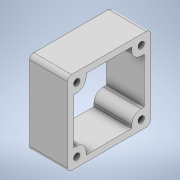
# Autodesk Inventor part: encoder_cover
Saved by Autodesk Inventor 2021 (Build 250183000, 183)
## iProperties
Created: 2021-01-13
Part Number: encoder_cover
Material: Generic
Document SubType Name: Modeling
Designer: Mateusz
Density: 1 g/cm^3
Appearance: Default
Author: Mateusz
Autodesk Inventor part; units mm, degrees
ref_plane "YZ Plane" through (0, 0, 0) normal (1, 0, 0) x (0, 1, 0)
ref_plane "XZ Plane" through (0, 0, 0) normal (0, 1, 0) x (-1, 0, 0)
ref_plane "XY Plane" through (0, 0, 0) normal (0, 0, 1) x (1, 0, 0)
sketch "Sketch1" plane through (0, 0, 0) normal (1, 0, 0) x (0, 1, 0)
  circle A0 centre (0, 0) radius 1.45
  circle A1 centre (0, -31) radius 1.45
  circle A2 centre (-31, -31) radius 1.45
  circle A3 centre (-31, 0) radius 1.45
  line L0 (0, 4.5) -> (-31, 4.5)
  line L1 (-31, 4.5) -> (-35.5, 4.5)
  line L2 (-35.5, 4.5) -> (-35.5, -35.5)
  line L3 (-35.5, -35.5) -> (4.5, -35.5)
  line L4 (4.5, -35.5) -> (4.5, 4.5)
  line L5 (4.5, 4.5) -> (0, 4.5)
  arc A4 (-4.5, 0) -> (0, -4.5) centre (0, 0) ccw
  arc A5 (-26.5, -31) -> (-31, -26.5) centre (-31, -31) ccw
  line L6 (-26.5, 0) -> (-26.5, 1.5)
  line L7 (-31, -4.5) -> (-32.5, -4.5)
  line L8 (-31, -26.5) -> (-32.5, -26.5)
  line L9 (-26.5, -31) -> (-26.5, -32.5)
  line L10 (-4.5, -31) -> (-4.5, -32.5)
  line L11 (0, -26.5) -> (1.5, -26.5)
  line L12 (0, -4.5) -> (1.5, -4.5)
  line L13 (-4.5, 0) -> (-4.5, 1.5)
  arc A6 (0, -26.5) -> (-4.5, -31) centre (0, -31) ccw
  arc A7 (-31, -4.5) -> (-26.5, 0) centre (-31, 0) ccw
  line L14 (-26.5, 1.5) -> (-4.5, 1.5)
  line L15 (1.5, -4.5) -> (1.5, -26.5)
  line L16 (-4.5, -32.5) -> (-26.5, -32.5)
  line L17 (-32.5, -26.5) -> (-32.5, -4.5)
  constraints: 36 end point, 14 perpendicular, 9 tangent, 8 centre point, 8 point on circle, 5 coincident, 3 point on line, 1 horizontal
extrude "Extrusion1" add sketch "Sketch1" along normal blind 18.2
fillet "Fillet1" radius 2 4 edges at (9.1, 4.5, 4.5) (9.1, 4.5, -35.5) (9.1, -35.5, 4.5) (9.1, -35.5, -35.5)
sketch "Sketch2" plane through (18.2, 0, 0) normal (1, 0, 0) x (0, 0, -1)
  circle A0 centre (0, 0) radius 1.45 projected
  circle A1 centre (0, 0) radius 1.525
  circle A2 centre (31, 0) radius 1.45 projected
  circle A3 centre (31, 0) radius 1.525
  circle A4 centre (31, -31) radius 1.45 projected
  circle A5 centre (31, -31) radius 1.525
  circle A6 centre (0, -31) radius 1.45 projected
  circle A7 centre (0, -31) radius 1.525
  dimension "d20" = 3.05
  dimension "d21" = 3.05
  dimension "d22" = 3.05
  dimension "d23" = 3.05
  constraints: 4 centre point, 4 coincident
  measures "d20" diameter of A1
  measures "d21" diameter of A3
  measures "d22" diameter of A5
  measures "d23" diameter of A7
extrude "Extrusion2" cut sketch "Sketch2" against normal up to surface (18.2 mm away)
body "Solid1"
